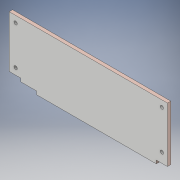
# Autodesk Inventor part: FP_PCB
Saved by Autodesk Inventor 2019 (Build 230136000, 136)
## iProperties
Created: 2020-09-16
Part Number: FP_PCB
Material: Generic
Document SubType Name: Modeling
Designer: johnh
Density: 1 g/cm^3
Appearance: Default
Author: johnh
Autodesk Inventor part; units mm, degrees
ref_plane "YZ Plane" through (0, 0, 0) normal (1, 0, 0) x (0, 1, 0)
ref_plane "XZ Plane" through (0, 0, 0) normal (0, 1, 0) x (-1, 0, 0)
ref_plane "XY Plane" through (0, 0, 0) normal (0, 0, 1) x (1, 0, 0)
sketch "Sketch1" plane through (0, 0, 0) normal (0, 0, 1) x (1, 0, 0)
  line L0 (15.0622, 60.5663) -> (170.4927, 60.5663)
  line L1 (170.4927, 60.5663) -> (170.4927, 9.7663)
  line L2 (15.0622, 9.7663) -> (15.0622, 60.5663)
  line L3 (170.4927, 9.7663) -> (170.4927, 6.5913)
  line L4 (26.4922, 6.5913) -> (26.4922, 9.7663)
  line L5 (159.5247, 6.5913) -> (159.5247, 3.4163)
  line L6 (159.5247, 3.4163) -> (42.0497, 3.4163)
  line L7 (42.0497, 3.4163) -> (42.0497, 6.5913)
  circle A0 centre (21.4122, 54.2163) radius 1.651
  circle A1 centre (21.4122, 16.129) radius 1.651
  circle A2 centre (165.0087, 16.129) radius 1.651
  circle A3 centre (165.0087, 54.2163) radius 1.651
  line L8 (33.3756, 50.5714) -> (117.4496, 50.5714)
  line L9 (117.4496, 50.5714) -> (117.4496, 28.8544)
  line L10 (117.4496, 28.8544) -> (33.3756, 28.8544)
  line L11 (33.3756, 28.8544) -> (33.3756, 50.5714)
  line L12 (39.2811, 23.114) -> (50.0761, 23.114)
  line L13 (50.0761, 23.114) -> (50.0761, 12.319)
  line L14 (50.0761, 12.319) -> (39.2811, 12.319)
  line L15 (39.2811, 12.319) -> (39.2811, 23.114)
  line L16 (54.6481, 23.114) -> (65.4431, 23.114)
  line L17 (65.4431, 23.114) -> (65.4431, 12.319)
  line L18 (65.4431, 12.319) -> (54.6481, 12.319)
  line L19 (54.6481, 12.319) -> (54.6481, 23.114)
  line L20 (70.0151, 23.114) -> (80.8101, 23.114)
  line L21 (80.8101, 23.114) -> (80.8101, 12.319)
  line L22 (80.8101, 12.319) -> (70.0151, 12.319)
  line L23 (70.0151, 12.319) -> (70.0151, 23.114)
  line L24 (85.3821, 23.114) -> (96.1771, 23.114)
  line L25 (96.1771, 23.114) -> (96.1771, 12.319)
  line L26 (96.1771, 12.319) -> (85.3821, 12.319)
  line L27 (85.3821, 12.319) -> (85.3821, 23.114)
  line L28 (100.7491, 23.114) -> (111.5441, 23.114)
  line L29 (111.5441, 23.114) -> (111.5441, 12.319)
  line L30 (111.5441, 12.319) -> (100.7491, 12.319)
  line L31 (100.7491, 12.319) -> (100.7491, 23.114)
  line L32 (138.7221, 23.114) -> (149.5171, 23.114)
  line L33 (149.5171, 23.114) -> (149.5171, 12.319)
  line L34 (149.5171, 12.319) -> (138.7221, 12.319)
  line L35 (138.7221, 12.319) -> (138.7221, 23.114)
  line L36 (170.4927, 9.7663) -> (170.4927, 9.7663)
  line L37 (26.4922, 9.7663) -> (15.0622, 9.7663)
  line L38 (26.4922, 6.5913) -> (42.0497, 6.5913)
  line L39 (159.5247, 6.5913) -> (170.4927, 6.5913)
  circle A4 centre (144.1196, 41.5163) radius 3.4925
  line L40 (144.1196, 23.114) -> (144.1196, 12.319)
  circle A5 centre (44.6786, 17.7165) radius 5.3975
  circle A6 centre (60.0456, 17.7165) radius 5.3975
  circle A7 centre (75.4126, 17.7165) radius 5.3975
  circle A8 centre (90.7796, 17.7165) radius 5.3975
  circle A9 centre (106.1466, 17.7165) radius 5.3975
  circle A10 centre (144.1196, 17.7165) radius 5.3975
  dimension "d0" = 3.302
  dimension "d1" = 6.35
  dimension "d2" = 6.35
  dimension "d3" = 84.074
  dimension "d4" = 21.717
  dimension "d5" = 10.795
  dimension "d6" = 10.795
  dimension "d7" = 10.795
  dimension "d8" = 10.795
  dimension "d9" = 10.795
  dimension "d10" = 10.795
  dimension "d11" = 10.795
  dimension "d12" = 4.572
  dimension "d13" = 4.572
  dimension "d14" = 4.572
  dimension "d15" = 4.572
  dimension "d16" = 5.9055
  dimension "d17" = 5.9055
  dimension "d21" = 6.985
  dimension "d22" = 26.67
  dimension "d25" = 0
  dimension "d26" = 3.302
  dimension "d28" = 3.302
  dimension "d32" = 50.8
  dimension "d33" = 155.4305
  dimension "d34" = 6.35
  dimension "d39" = 26.373
  dimension "d40" = 19.05
  dimension "d41" = 29.6164
  dimension "d43" = 15.367
  dimension "d44" = 37.973
  constraints: 82 end point, 17 parallel, 11 centre point, 10 horizontal, 10 point on line, 8 perpendicular, 3 midpoint, 2 collinear, 1 tangent
  measures "d0" diameter of A0
  measures "d1" distance from line of L0 A0.centre
  measures "d2" distance from line of A0.centre L2
  measures "d3" distance of L9.end L10.end
  measures "d4" distance of L8.end L9.end
  measures "d5" distance of L13.end L14.end
  measures "d6" distance of L12.end L13.end
  measures "d7" distance of L17.end L18.end
  measures "d8" distance of L21.end L22.end
  measures "d9" distance of L25.end L26.end
  measures "d10" distance of L29.end L30.end
  measures "d11" distance of L33.end L34.end
  measures "d12" distance between parallel lines of L19 L13
  measures "d13" distance between parallel lines of L23 L17
  measures "d14" distance between parallel lines of L27 L21
  measures "d15" distance between parallel lines of L31 L25
  measures "d16" distance between parallel lines of L9 L29
  measures "d17" distance between parallel lines of L11 L15
  measures "d21" diameter of A4
  measures "d22" distance from line of A4.centre L9
  measures "d25" distance from line of A4.centre L40
  measures "d26" diameter of A3
  measures "d28" diameter of A1
  measures "d32" distance of L2.start L0.start
  measures "d33" distance of L0.start L0.end
  measures "d34" distance between parallel lines of L6 L37
  measures "d39" distance from line of L1 A4.centre
  measures "d40" distance from line of L0 A4.centre
  measures "d41" distance from line of L2 A5.centre
  measures "d43" distance of A6.centre A5.centre
  measures "d44" distance of A10.centre A9.centre
sketch "Sketch2" plane through (0, 0, 0) normal (0, 0, 1) x (1, 0, 0)
  line L0 (15.0622, 9.7663) -> (15.0622, 60.5663) projected
  line L1 (15.0622, 60.5663) -> (170.4927, 60.5663) projected
  line L2 (33.3756, 50.5714) -> (117.4496, 50.5714) projected
  line L3 (117.4496, 50.5714) -> (117.4496, 28.8544) projected
  line L4 (170.4927, 60.5663) -> (170.4927, 9.7663) projected
  line L5 (159.5247, 6.5913) -> (170.4927, 6.5913) projected
  line L6 (159.5247, 6.5913) -> (159.5247, 3.4163) projected
  line L7 (159.5247, 3.4163) -> (42.0497, 3.4163) projected
  line L8 (42.0497, 3.4163) -> (42.0497, 6.5913) projected
  line L9 (26.4922, 6.5913) -> (42.0497, 6.5913) projected
  line L10 (26.4922, 6.5913) -> (26.4922, 9.7663) projected
  line L11 (26.4922, 9.7663) -> (15.0622, 9.7663) projected
  circle A0 centre (21.4122, 16.129) radius 1.651 projected
  circle A1 centre (21.4122, 54.2163) radius 1.651 projected
  circle A2 centre (165.0087, 54.2163) radius 1.651 projected
  circle A3 centre (165.0087, 16.129) radius 1.651 projected
  line L12 (15.0622, 60.5663) -> (15.0622, 9.7663)
  line L13 (15.0622, 9.7663) -> (26.4922, 9.7663)
  line L14 (26.4922, 9.7663) -> (26.4922, 6.5913)
  line L15 (26.4922, 6.5913) -> (42.0497, 6.5913)
  line L16 (42.0497, 6.5913) -> (42.0497, 3.4163)
  line L17 (42.0497, 3.4163) -> (159.5247, 3.4163)
  line L18 (159.5247, 3.4163) -> (159.5247, 6.5913)
  line L19 (159.5247, 6.5913) -> (170.4927, 6.5913)
  line L20 (170.4927, 6.5913) -> (170.4927, 60.5663)
  line L21 (170.4927, 60.5663) -> (15.0622, 60.5663)
  circle A4 centre (21.4122, 54.2163) radius 1.651
  circle A5 centre (21.4122, 16.129) radius 1.651
  circle A6 centre (165.0087, 16.129) radius 1.651
  circle A7 centre (165.0087, 54.2163) radius 1.651
  point P0 (0, 0)
  point P1 (144.1196, 41.5163)
  constraints: 20 end point, 6 perpendicular, 4 centre point, 4 coincident, 4 collinear, 4 concentric
surface extrude "ExtrusionSrf1" sketch "Sketch1" along normal blind 3.302 shown yes curves L0 L1 L36 L3 L39 L5 L6 L7 L38 L4 L37 L2
extrude "Extrusion1" add sketch "Sketch2" along normal blind 3.302
equation "\"d35\" = d28"
equation "\"d37\" = d28"
body "Solid1"
body "Srf1"
